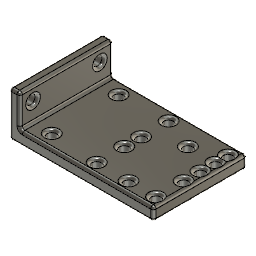
Microswitch Mount_L (Autodesk Fusion 360 design; units mm, degrees)
Autodesk Fusion 360 part; units mm, degrees
note: some values were not read from the file. Set by a fixed rule: which sketch regions a step uses.
sketch "Sketch1" plane through (0, 0, 0) normal (0, 1, 0) x (1, 0, 0)
  line L0 (6.5, 6.5) -> (-6.5, 6.5)
  line L1 (-6.5, -6.5) -> (6.5, 6.5) construction
  line L2 (6.5, -6.5) -> (-6.5, 6.5) construction
  line L3 (-0.5, 9.5) -> (-9.5, 9.5)
  line L4 (-0.5, -9.5) -> (-0.5, 9.5)
  line L5 (-5.5, 4.5) -> (44.5, 4.5)
  line L6 (44.5, 4.5) -> (44.5, 9.5)
  line L7 (44.5, 9.5) -> (-5.5, 9.5)
  line L8 (-5.5, 9.5) -> (-5.5, 4.5)
  line L9 (-5.5, 9.5) -> (-9.5, 9.5)
  line L10 (-9.5, 9.5) -> (-9.5, -7.5)
  line L11 (-9.5, -7.5) -> (-5.5, -7.5)
  line L12 (-5.5, -7.5) -> (-5.5, 9.5)
  dimension "d1" = 13
  dimension "d2" = 13
  dimension "d6" = 5
  dimension "d39" = 4
  dimension "d40" = 12
  dimension "d49" = 50
  constraint horizontal L5
  constraint vertical L6
  constraint horizontal L7
  constraint vertical L8
  constraint collinear L3 L7
  constraint horizontal L9
  constraint vertical L10
  constraint horizontal L11
  constraint vertical L12
  measures "d1" distance of L0.start L0.end
  measures "d2" distance of L2.start L0.start
  measures "d6" distance of L5 L7
  measures "d39" distance of L7.end L3.end
  measures "d40" distance of L5 L11
  measures "d49" distance of L6 L12
extrude "Extrude1" add sketch "Sketch1" along normal blind 35 contours L0 L4 L5 L8 L12 | L4 L5 L6 L7 | L0 L3 L4 L7 L8 L12 | L3 L8 L9 L10 L11 L12
sketch "Sketch2" plane through (0, 0, -4.5) normal (0, 0, 1) x (-1, 0, 0)
  line L0 (9.5, 0) -> (-16.5, 0)
  line L1 (-16.5, 0) -> (-16.5, -35)
  line L2 (-16.5, -35) -> (9.5, -35)
  line L3 (9.5, -35) -> (9.5, 0)
  circle A0 centre (-1.5, -5) radius 1.8
  circle A1 centre (-1.5, -30) radius 1.8
  circle A2 centre (-41.5, -4) radius 1.8
  line L4 (-44.5, 0) -> (-44.5, -35)
  line L5 (-6.5, 0) -> (-44.5, 0)
  circle A3 centre (-19.3, -4) radius 1.8
  circle A4 centre (-41.5, -14.3) radius 1.8
  circle A5 centre (-19.3, -14.3) radius 1.8
  circle A6 centre (-41.5, -30.9) radius 1.8
  circle A7 centre (-19.3, -20.6) radius 1.8
  circle A8 centre (-41.5, -20.6) radius 1.8
  circle A9 centre (-19.3, -30.9) radius 1.8
  circle A10 centre (-41.5, -26.2) radius 1.8
  circle A11 centre (-31.2, -4) radius 1.8
  circle A12 centre (-31.2, -26.2) radius 1.8
  line L6 (5.5, 0) -> (-44.5, 0)
  line L7 (-44.5, 0) -> (-44.5, -35)
  line L8 (-44.5, -35) -> (5.5, -35)
  line L9 (5.5, -35) -> (5.5, 0)
  dimension "d14" = 3.6
  dimension "d15" = 3.6
  dimension "d16" = 15
  dimension "d17" = 5
  dimension "d18" = 15
  dimension "d19" = 5
  dimension "d20" = 3.6
  dimension "d21" = 3
  dimension "d22" = 4
  dimension "d25" = -22.2
  dimension "d26" = 10.3
  dimension "d29" = 16.6
  dimension "d30" = 0
  dimension "d33" = 22.2
  dimension "d34" = 10.3
  measures "d14" diameter of A0
  measures "d15" diameter of A1
  measures "d16" distance of L1 A1.centre
  measures "d17" distance of L2 A1.centre
  measures "d18" distance of L1 A0.centre
  measures "d19" distance of L0 A0.centre
  measures "d20" diameter of A2
  measures "d21" distance of A2.centre L4
  measures "d22" distance of A2.centre L5
extrude "Extrude2" cut sketch "Sketch2" against normal up to surface (5 mm away) contours A0 | A1 | A2 | A3 | A4 | A5 | A6 | A7 | A8 | A9 | A10 | A11 | A12
sketch "Sketch3" plane through (-5.5, 0, 0) normal (1, 0, 0) x (0, 1, 0)
  line L0 (0, 7.5) -> (0, -4.5)
  line L1 (0, -4.5) -> (35, -4.5)
  line L2 (35, -4.5) -> (35, 7.5)
  line L3 (35, 7.5) -> (0, 7.5)
  circle A0 centre (5, 2.5) radius 1.75
  circle A1 centre (30, 2.5) radius 1.75
  dimension "d41" = 3.5
  dimension "d42" = 3.5
  dimension "d43" = 5
  dimension "d44" = 5
  dimension "d45" = 5
  dimension "d46" = 5
  measures "d41" diameter of A0
  measures "d42" diameter of A1
  measures "d43" distance of L3 A0.centre
  measures "d44" distance of L0 A0.centre
  measures "d45" distance of L3 A1.centre
  measures "d46" distance of L2 A1.centre
extrude "Extrude3" cut sketch "Sketch3" against normal blind 5 contours A0 | A1
fillet "Fillet2" radius 1 3 edges at (44.5, 0, -7) (44.5, 35, -7) (43.1782, 31.5509, -9.5) 18 faces at (-0.2978, 30.0897, -7.8333) (-0.2978, 5.0897, -7.8333) (17.5022, 30.9897, -7.8333) (29.4022, 26.2897, -7.8333) (42.691, 32.2496, -7.8333) (39.7022, 26.2897, -7.8333) (39.7022, 20.6897, -7.8333) (17.5022, 20.6897, -7.8333) (17.5022, 14.3897, -7.8333) (17.5022, 4.0897, -7.8333) (29.4022, 4.0897, -7.8333) (39.7022, 4.0897, -7.8333) (39.7022, 14.3897, -7.8333) (7.2984, 18.3565, -4.5) (-5.5, 21.375, -2.6718) (7.2984, 18.3565, -9.5) (-8.1667, 23.3333, 7.5) (-9.5, 13.697, -5.9561)
